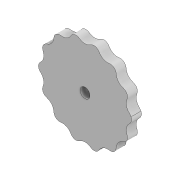
# Autodesk Inventor part: hypocycloid_Disk
Saved by Autodesk Inventor 2022 (Build 260153000, 153)
## iProperties
Created: 2023-10-31
Part Number: hypocycloid_Disk
Material: 一般
Document SubType Name: Modeling
Designer: JOU
Density: 1 g/cm^3
Appearance: 預設
Author: JOU
Autodesk Inventor part; units mm, degrees
ref_plane "YZ Plane" through (0, 0, 0) normal (1, 0, 0) x (0, 1, 0)
ref_plane "XZ Plane" through (0, 0, 0) normal (0, 1, 0) x (-1, 0, 0)
ref_plane "XY Plane" through (0, 0, 0) normal (0, 0, 1) x (1, 0, 0)
sketch "草圖1" plane through (0, 0, 0) normal (0, 0, 1) x (1, 0, 0)
  spline S0 degree 3 poles (46.5081, 2.287) (46.2704, 2.7291) (45.8908, 3.4351) (45.2157, 4.1892) (44.7361, 4.6818) (44.3407, 5.0888) (43.9753, 5.4923) (43.6176, 5.9301) (43.2647, 6.4206) (42.9232, 6.9706) (42.6037, 7.5793) (42.318, 8.2402) (42.0769, 8.9423) (41.8889, 9.6714) (41.7589, 10.4112) (41.6883, 11.145) (41.6748, 11.8565) (41.7124, 12.5321) (41.7927, 13.1621) (41.9064, 13.7433) (42.0452, 14.2825) (42.2058, 14.8031) (42.3946, 15.3604) (42.63, 16.0764) (42.9005, 17.197) (42.9458, 18.9694) (42.1848, 21.0267) (40.7738, 22.4576) (39.5432, 23.1408) (38.7166, 23.4695) (38.1155, 23.6851) (37.5969, 23.8798) (37.0926, 24.0926) (36.5754, 24.3448) (36.0395, 24.6496) (35.4903, 25.0146) (34.9391, 25.4423) (34.3999, 25.9307) (33.887, 26.4733) (33.4138, 27.0599) (32.991, 27.6774) (32.6262, 28.3108) (32.323, 28.9446) (32.0809, 29.5642) (31.8955, 30.1587) (31.7586, 30.7231) (31.6591, 31.264) (31.5829, 31.8082) (31.5089, 32.4228) (31.3878, 33.2528) (31.0541, 34.5283) (30.0978, 36.2136) (28.3292, 37.5348) (26.5257, 37.9827) (25.2925, 37.9927) (24.5019, 37.9235) (23.9028, 37.8611) (23.3579, 37.8174) (22.8052, 37.7979) (22.2189, 37.811) (21.5924, 37.866) (20.9298, 37.9719) (20.2416, 38.1349) (19.5423, 38.3583) (18.8479, 38.6414) (18.1747, 38.9797) (17.5376, 39.3651) (16.949, 39.7865) (16.4179, 40.2312) (15.9488, 40.6861) (15.5409, 41.1401) (15.1869, 41.5872) (14.8714, 42.0321) (14.5648, 42.5005) (14.2079, 43.0575) (13.6627, 43.8308) (12.6288, 44.9164) (10.8089, 45.908) (8.6482, 46.0552) (7.0352, 45.5727) (6.0788, 45.0757) (5.4648, 44.7021) (4.9727, 44.4012) (4.4999, 44.1319) (3.9995, 43.8786) (3.4506, 43.641) (2.8463, 43.4263) (2.1888, 43.2447) (1.4864, 43.1063) (0.7516, 43.0196) (0, 42.9901) (-0.7516, 43.0196) (-1.4864, 43.1063) (-2.1888, 43.2447) (-2.8463, 43.4263) (-3.4506, 43.641) (-3.9995, 43.8786) (-4.4999, 44.1319) (-4.9727, 44.4012) (-5.4648, 44.7021) (-6.0788, 45.0757) (-7.0352, 45.5727) (-8.6482, 46.0552) (-10.8089, 45.908) (-12.6288, 44.9164) (-13.6627, 43.8308) (-14.2079, 43.0575) (-14.5648, 42.5005) (-14.8714, 42.0321) (-15.1869, 41.5872) (-15.5409, 41.1401) (-15.9488, 40.6861) (-16.4179, 40.2312) (-16.949, 39.7865) (-17.5376, 39.3651) (-18.1747, 38.9797) (-18.8479, 38.6414) (-19.5423, 38.3583) (-20.2416, 38.1349) (-20.9298, 37.9719) (-21.5924, 37.866) (-22.2189, 37.811) (-22.8052, 37.7979) (-23.3579, 37.8174) (-23.9028, 37.8611) (-24.5019, 37.9235) (-25.2925, 37.9927) (-26.5257, 37.9827) (-28.3292, 37.5348) (-30.0978, 36.2136) (-31.0541, 34.5283) (-31.3878, 33.2528) (-31.5089, 32.4228) (-31.5829, 31.8082) (-31.6591, 31.264) (-31.7586, 30.7231) (-31.8955, 30.1587) (-32.0809, 29.5642) (-32.323, 28.9446) (-32.6262, 28.3108) (-32.991, 27.6774) (-33.4138, 27.0599) (-33.887, 26.4733) (-34.3999, 25.9307) (-34.9391, 25.4423) (-35.4903, 25.0146) (-36.0395, 24.6496) (-36.5754, 24.3448) (-37.0926, 24.0926) (-37.5969, 23.8798) (-38.1155, 23.6851) (-38.7166, 23.4695) (-39.5432, 23.1408) (-40.7738, 22.4576) (-42.1848, 21.0267) (-42.9458, 18.9694) (-42.9005, 17.197) (-42.63, 16.0764) (-42.3946, 15.3604) (-42.2058, 14.8031) (-42.0452, 14.2825) (-41.9064, 13.7433) (-41.7927, 13.1621) (-41.7124, 12.5321) (-41.6748, 11.8565) (-41.6883, 11.145) (-41.7589, 10.4112) (-41.8889, 9.6714) (-42.0769, 8.9423) (-42.318, 8.2402) (-42.6037, 7.5793) (-42.9232, 6.9706) (-43.2647, 6.4206) (-43.6176, 5.9301) (-43.9752, 5.4923) (-44.3407, 5.0888) (-44.7358, 4.6817) (-45.217, 4.1898) (-45.8816, 3.4306) (-46.7163, 2.0754) (-47.1729, 0) (-46.7163, -2.0754) (-45.8816, -3.4306) (-45.217, -4.1898) (-44.7358, -4.6817) (-44.3407, -5.0888) (-43.9752, -5.4923) (-43.6176, -5.9301) (-43.2647, -6.4206) (-42.9232, -6.9706) (-42.6037, -7.5793) (-42.318, -8.2402) (-42.0769, -8.9423) (-41.8889, -9.6714) (-41.7589, -10.4112) (-41.6883, -11.145) (-41.6748, -11.8565) (-41.7124, -12.5321) (-41.7927, -13.1621) (-41.9064, -13.7433) (-42.0452, -14.2825) (-42.2058, -14.8031) (-42.3946, -15.3604) (-42.63, -16.0764) (-42.9005, -17.197) (-42.9458, -18.9694) (-42.1848, -21.0267) (-40.7738, -22.4576) (-39.5432, -23.1408) (-38.7166, -23.4695) (-38.1155, -23.6851) (-37.5969, -23.8798) (-37.0926, -24.0926) (-36.5754, -24.3448) (-36.0395, -24.6496) (-35.4903, -25.0146) (-34.9391, -25.4423) (-34.3999, -25.9307) (-33.887, -26.4733) (-33.4138, -27.0599) (-32.991, -27.6774) (-32.6262, -28.3108) (-32.323, -28.9446) (-32.0809, -29.5642) (-31.8955, -30.1587) (-31.7586, -30.7231) (-31.6591, -31.264) (-31.5829, -31.8082) (-31.5089, -32.4228) (-31.3878, -33.2528) (-31.0541, -34.5283) (-30.0978, -36.2136) (-28.3292, -37.5348) (-26.5257, -37.9827) (-25.2925, -37.9927) (-24.5019, -37.9235) (-23.9028, -37.8611) (-23.3579, -37.8174) (-22.8052, -37.7979) (-22.2189, -37.811) (-21.5924, -37.866) (-20.9298, -37.9719) (-20.2416, -38.1349) (-19.5423, -38.3583) (-18.8479, -38.6414) (-18.1747, -38.9797) (-17.5376, -39.3651) (-16.949, -39.7865) (-16.4179, -40.2312) (-15.9488, -40.6861) (-15.5409, -41.1401) (-15.1869, -41.5872) (-14.8714, -42.0321) (-14.5648, -42.5005) (-14.2079, -43.0575) (-13.6627, -43.8308) (-12.6288, -44.9164) (-10.8089, -45.908) (-8.6482, -46.0552) (-7.0352, -45.5727) (-6.0788, -45.0757) (-5.4648, -44.7021) (-4.9727, -44.4012) (-4.4999, -44.1319) (-3.9995, -43.8786) (-3.4506, -43.641) (-2.8463, -43.4263) (-2.1888, -43.2447) (-1.4864, -43.1063) (-0.7516, -43.0196) (0, -42.9901) (0.7516, -43.0196) (1.4864, -43.1063) (2.1888, -43.2447) (2.8463, -43.4263) (3.4506, -43.641) (3.9995, -43.8786) (4.4999, -44.1319) (4.9727, -44.4012) (5.4648, -44.7021) (6.0788, -45.0757) (7.0352, -45.5727) (8.6482, -46.0552) (10.8089, -45.908) (12.6288, -44.9164) (13.6627, -43.8308) (14.2079, -43.0575) (14.5648, -42.5005) (14.8714, -42.0321) (15.1869, -41.5872) (15.5409, -41.1401) (15.9488, -40.6861) (16.4179, -40.2312) (16.949, -39.7865) (17.5376, -39.3651) (18.1747, -38.9797) (18.8479, -38.6414) (19.5423, -38.3583) (20.2416, -38.1349) (20.9298, -37.9719) (21.5924, -37.866) (22.2189, -37.811) (22.8052, -37.7979) (23.3579, -37.8174) (23.9028, -37.8611) (24.5019, -37.9235) (25.2925, -37.9927) (26.5257, -37.9827) (28.3292, -37.5348) (30.0978, -36.2136) (31.0541, -34.5283) (31.3878, -33.2528) (31.5089, -32.4228) (31.5829, -31.8082) (31.6591, -31.264) (31.7586, -30.7231) (31.8955, -30.1587) (32.0809, -29.5642) (32.323, -28.9446) (32.6262, -28.3108) (32.991, -27.6774) (33.4138, -27.0599) (33.887, -26.4733) (34.3999, -25.9307) (34.9391, -25.4423) (35.4903, -25.0146) (36.0395, -24.6496) (36.5754, -24.3448) (37.0926, -24.0926) (37.5969, -23.8798) (38.1155, -23.6851) (38.7166, -23.4695) (39.5432, -23.1408) (40.7738, -22.4576) (42.1848, -21.0267) (42.9458, -18.9694) (42.9005, -17.197) (42.63, -16.0764) (42.3946, -15.3604) (42.2058, -14.8031) (42.0452, -14.2825) (41.9064, -13.7433) (41.7927, -13.1621) (41.7124, -12.5321) (41.6748, -11.8565) (41.6883, -11.145) (41.7589, -10.4112) (41.8889, -9.6714) (42.0769, -8.9423) (42.318, -8.2402) (42.6037, -7.5793) (42.9232, -6.9706) (43.2647, -6.4206) (43.6176, -5.9301) (43.9752, -5.4923) (44.3407, -5.0888) (44.7358, -4.6817) (45.2169, -4.1898) (45.8824, -3.4302) (46.7096, -2.0786) (47.2127, 0.0192) (46.743, 1.5311) (46.5081, 2.287) knots 0 0 0 0 0.149893 0.239343 0.302293 0.356324 0.409534 0.46556 0.525845 0.590663 0.659617 0.7319 0.806459 0.882095 0.95755 1.031576 1.103007 1.170847 1.234388 1.293389 1.348393 1.40133 1.456795 1.524916 1.627422 1.801794 2.049428 2.261874 2.390188 2.469404 2.528561 2.581789 2.635555 2.692715 2.754303 2.820366 2.890366 2.963415 3.038407 3.114121 3.189293 3.262691 3.333188 3.399856 3.462097 3.519855 3.573988 3.62701 3.684699 3.759705 3.878536 4.078589 4.329136 4.516357 4.626594 4.697919 4.754386 4.807316 4.861862 4.920235 4.983128 5.050389 5.121363 5.195087 5.270413 5.346101 5.420889 5.493566 5.563052 5.628497 5.689433 5.746013 5.79947 5.853029 5.913929 5.99794 6.136622 6.360535 6.602519 6.764364 6.85996 6.925304 6.979964 7.032997 7.088496 7.148135 7.212319 7.280724 7.352591 7.426895 7.502454 7.578012 7.652317 7.724184 7.792589 7.856773 7.916412 7.97191 8.024944 8.079604 8.144948 8.240544 8.402389 8.644373 8.868286 9.006968 9.090979 9.151878 9.205438 9.258895 9.315475 9.376411 9.441856 9.511342 9.584019 9.658807 9.734495 9.809821 9.883545 9.954519 10.02178 10.084673 10.143046 10.197592 10.250522 10.306989 10.378314 10.488551 10.675772 10.926319 11.126372 11.245202 11.320208 11.377897 11.43092 11.485052 11.54281 11.605052 11.67172 11.742217 11.815614 11.890787 11.9665 12.041493 12.114542 12.184542 12.250604 12.312193 12.369352 12.423119 12.476347 12.535504 12.61472 12.743033 12.95548 13.203114 13.377486 13.479992 13.548113 13.603578 13.656515 13.711519 13.77052 13.834061 13.901901 13.973332 14.047358 14.122813 14.198449 14.273007 14.345291 14.414244 14.479063 14.539348 14.595374 14.648584 14.702615 14.765565 14.855015 15.004908 15.238836 15.472765 15.622657 15.712108 15.775058 15.829089 15.882299 15.938324 15.998609 16.063428 16.132382 16.204665 16.279223 16.354859 16.430315 16.50434 16.575771 16.643612 16.707153 16.766154 16.821158 16.874094 16.92956 16.99768 17.100187 17.274558 17.522192 17.734639 17.862953 17.942168 18.001325 18.054553 18.10832 18.165479 18.227068 18.29313 18.363131 18.43618 18.511172 18.586886 18.662058 18.735456 18.805952 18.87262 18.934862 18.99262 19.046752 19.099775 19.157464 19.23247 19.351301 19.551354 19.801901 19.989121 20.099358 20.170683 20.22715 20.28008 20.334627 20.393 20.455893 20.523154 20.594127 20.667851 20.743177 20.818865 20.893653 20.96633 21.035816 21.101262 21.162197 21.218778 21.272235 21.325794 21.386694 21.470704 21.609387 21.833299 22.075283 22.237129 22.332725 22.398068 22.452728 22.505762 22.56126 22.6209 22.685083 22.753488 22.825356 22.89966 22.975218 23.050777 23.125081 23.196949 23.265354 23.329537 23.389177 23.444675 23.497709 23.552369 23.617712 23.713308 23.875154 24.117138 24.34105 24.479733 24.563743 24.624643 24.678202 24.731659 24.78824 24.849175 24.914621 24.984107 25.056784 25.131572 25.207259 25.282586 25.356309 25.427283 25.494544 25.557437 25.61581 25.670357 25.723287 25.779754 25.851079 25.961316 26.148536 26.399083 26.599136 26.717967 26.792973 26.850662 26.903685 26.957817 27.015575 27.077817 27.144485 27.214981 27.288379 27.363551 27.439265 27.514257 27.587306 27.657307 27.723369 27.784958 27.842117 27.895884 27.949112 28.008269 28.087484 28.215798 28.428245 28.675878 28.85025 28.952757 29.020877 29.076343 29.129279 29.184283 29.243284 29.306825 29.374666 29.446097 29.520122 29.595578 29.671214 29.745772 29.818055 29.887009 29.951828 30.012113 30.068138 30.121348 30.175379 30.238329 30.32778 30.477672 30.711601 30.945529 30.945529 30.945529 30.945529
  point P0 (0, 0)
  point P1 (45.1518, 4.2496)
  point P2 (44.7153, 4.7032)
  point P3 (44.3411, 5.0929)
  point P4 (43.9849, 5.4882)
  point P5 (43.6309, 5.9225)
  point P6 (43.279, 6.412)
  point P7 (42.937, 6.9626)
  point P8 (42.6165, 7.5731)
  point P9 (42.3296, 8.2366)
  point P10 (42.0874, 8.9417)
  point P11 (41.8984, 9.6741)
  point P12 (41.7679, 10.4173)
  point P13 (41.6971, 11.1541)
  point P14 (41.6836, 11.8683)
  point P15 (41.7214, 12.5457)
  point P16 (41.8018, 13.176)
  point P17 (41.9148, 13.7551)
  point P18 (42.0512, 14.2879)
  point P19 (42.2056, 14.7943)
  point P20 (42.3804, 15.3207)
  point P21 (42.5872, 15.9697)
  point P22 (42.8177, 16.9685)
  point P23 (42.8468, 18.712)
  point P24 (41.9828, 21.0327)
  point P25 (40.5015, 22.5556)
  point P26 (39.3859, 23.1894)
  point P27 (38.6527, 23.4894)
  point P28 (38.0974, 23.6933)
  point P29 (37.5999, 23.8825)
  point P30 (37.1049, 24.0925)
  point P31 (36.5914, 24.3435)
  point P32 (36.0561, 24.6481)
  point P33 (35.5059, 25.0137)
  point P34 (34.9528, 25.4427)
  point P35 (34.4112, 25.933)
  point P36 (33.896, 26.478)
  point P37 (33.4207, 27.0672)
  point P38 (32.9961, 27.6876)
  point P39 (32.6298, 28.3236)
  point P40 (32.3257, 28.9596)
  point P41 (32.0832, 29.5806)
  point P42 (31.8977, 30.1748)
  point P43 (31.7612, 30.736)
  point P44 (31.6623, 31.2682)
  point P45 (31.5867, 31.793)
  point P46 (31.5137, 32.3653)
  point P47 (31.3983, 33.1064)
  point P48 (31.0861, 34.253)
  point P49 (30.0855, 35.9853)
  point P50 (28.0793, 37.4861)
  point P51 (26.2661, 37.9525)
  point P52 (25.1639, 37.9725)
  point P53 (24.4528, 37.917)
  point P54 (23.8908, 37.8622)
  point P55 (23.363, 37.8217)
  point P56 (22.8179, 37.8034)
  point P57 (22.2343, 37.8168)
  point P58 (21.6078, 37.8719)
  point P59 (20.9436, 37.9779)
  point P60 (20.2529, 38.1414)
  point P61 (19.5506, 38.3656)
  point P62 (18.8531, 38.6499)
  point P63 (18.1768, 38.9898)
  point P64 (17.5369, 39.3769)
  point P65 (16.9461, 39.8001)
  point P66 (16.4134, 40.2464)
  point P67 (15.9436, 40.702)
  point P68 (15.5362, 41.1551)
  point P69 (15.1846, 41.5984)
  point P70 (14.8743, 42.0337)
  point P71 (14.5789, 42.4805)
  point P72 (14.2463, 42.9906)
  point P73 (13.7554, 43.6724)
  point P74 (12.7892, 44.6673)
  point P75 (10.8168, 45.7271)
  point P76 (8.4032, 45.8999)
  point P77 (6.8484, 45.4503)
  point P78 (5.9957, 45.0182)
  point P79 (5.4345, 44.6834)
  point P80 (4.9666, 44.4008)
  point P81 (4.505, 44.1397)
  point P82 (4.0096, 43.8897)
  point P83 (3.4621, 43.653)
  point P84 (2.8573, 43.4381)
  point P85 (2.198, 43.2559)
  point P86 (1.4929, 43.1169)
  point P87 (0.755, 43.0297)
  point P88 (0, 43)
  point P89 (-0.755, 43.0297)
  point P90 (-1.4929, 43.1169)
  point P91 (-2.198, 43.2559)
  point P92 (-2.8573, 43.4381)
  point P93 (-3.4621, 43.653)
  point P94 (-4.0096, 43.8897)
  point P95 (-4.505, 44.1397)
  point P96 (-4.9666, 44.4008)
  point P97 (-5.4345, 44.6834)
  point P98 (-5.9957, 45.0182)
  point P99 (-6.8484, 45.4503)
  point P100 (-8.4032, 45.8999)
  point P101 (-10.8168, 45.7271)
  point P102 (-12.7892, 44.6673)
  point P103 (-13.7554, 43.6724)
  point P104 (-14.2463, 42.9906)
  point P105 (-14.5789, 42.4805)
  point P106 (-14.8743, 42.0337)
  point P107 (-15.1846, 41.5984)
  point P108 (-15.5362, 41.1551)
  point P109 (-15.9436, 40.702)
  point P110 (-16.4134, 40.2464)
  point P111 (-16.9461, 39.8001)
  point P112 (-17.5369, 39.3769)
  point P113 (-18.1768, 38.9898)
  point P114 (-18.8531, 38.6499)
  point P115 (-19.5506, 38.3656)
  point P116 (-20.2529, 38.1414)
  point P117 (-20.9436, 37.9779)
  point P118 (-21.6078, 37.8719)
  point P119 (-22.2343, 37.8168)
  point P120 (-22.8179, 37.8034)
  point P121 (-23.363, 37.8217)
  point P122 (-23.8908, 37.8622)
  point P123 (-24.4528, 37.917)
  point P124 (-25.1639, 37.9725)
  point P125 (-26.2661, 37.9525)
  point P126 (-28.0793, 37.4861)
  point P127 (-30.0855, 35.9853)
  point P128 (-31.0861, 34.253)
  point P129 (-31.3983, 33.1064)
  point P130 (-31.5137, 32.3653)
  point P131 (-31.5867, 31.793)
  point P132 (-31.6623, 31.2682)
  point P133 (-31.7612, 30.736)
  point P134 (-31.8977, 30.1748)
  point P135 (-32.0832, 29.5806)
  point P136 (-32.3257, 28.9596)
  point P137 (-32.6298, 28.3236)
  point P138 (-32.9961, 27.6876)
  point P139 (-33.4207, 27.0672)
  point P140 (-33.896, 26.478)
  point P141 (-34.4112, 25.933)
  point P142 (-34.9528, 25.4427)
  point P143 (-35.5059, 25.0137)
  point P144 (-36.0561, 24.6481)
  point P145 (-36.5914, 24.3435)
  point P146 (-37.1049, 24.0925)
  point P147 (-37.5999, 23.8825)
  point P148 (-38.0974, 23.6933)
  point P149 (-38.6527, 23.4894)
  point P150 (-39.3859, 23.1894)
  point P151 (-40.5015, 22.5556)
  point P152 (-41.9828, 21.0327)
  point P153 (-42.8468, 18.712)
  point P154 (-42.8177, 16.9685)
  point P155 (-42.5872, 15.9697)
  point P156 (-42.3804, 15.3207)
  point P157 (-42.2056, 14.7943)
  point P158 (-42.0512, 14.2879)
  point P159 (-41.9148, 13.7551)
  point P160 (-41.8018, 13.176)
  point P161 (-41.7214, 12.5457)
  point P162 (-41.6836, 11.8683)
  point P163 (-41.6971, 11.1541)
  point P164 (-41.7679, 10.4173)
  point P165 (-41.8984, 9.6741)
  point P166 (-42.0874, 8.9417)
  point P167 (-42.3296, 8.2366)
  point P168 (-42.6165, 7.5731)
  point P169 (-42.937, 6.9626)
  point P170 (-43.279, 6.412)
  point P171 (-43.6309, 5.9225)
  point P172 (-43.9849, 5.4882)
  point P173 (-44.3411, 5.0929)
  point P174 (-44.7153, 4.7032)
  point P175 (-45.1518, 4.2496)
  point P176 (-45.7341, 3.5706)
  point P177 (-46.5081, 2.287)
  point P178 (-47, 0)
  point P179 (-46.5081, -2.287)
  point P180 (-45.7341, -3.5706)
  point P181 (-45.1518, -4.2496)
  point P182 (-44.7153, -4.7032)
  point P183 (-44.3411, -5.0929)
  point P184 (-43.9849, -5.4882)
  point P185 (-43.6309, -5.9225)
  point P186 (-43.279, -6.412)
  point P187 (-42.937, -6.9626)
  point P188 (-42.6165, -7.5731)
  point P189 (-42.3296, -8.2366)
  point P190 (-42.0874, -8.9417)
  point P191 (-41.8984, -9.6741)
  point P192 (-41.7679, -10.4173)
  point P193 (-41.6971, -11.1541)
  point P194 (-41.6836, -11.8683)
  point P195 (-41.7214, -12.5457)
  point P196 (-41.8018, -13.176)
  point P197 (-41.9148, -13.7551)
  point P198 (-42.0512, -14.2879)
  point P199 (-42.2056, -14.7943)
  constraints: 360 other
extrude "擠出1" add sketch "草圖1" along normal blind 10
sketch "草圖2" plane through (0, 0, 10) normal (0, 0, 1) x (1, 0, 0)
  circle A0 centre (0, 0) radius 5
  dimension "d2" = 10
  constraints: 1 centre point, 1 coincident
  measures "d2" diameter of A0
extrude "擠出2" cut sketch "草圖2" against normal up to next
